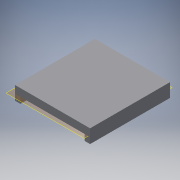
# Autodesk Inventor part: left gun mount
Saved by Autodesk Inventor 2018 (Build 220112000, 112)
## iProperties
Created: 2018-11-09
Part Number: left gun mount
Material: Generic
Document SubType Name: Modeling
Designer: Cameron
Mass: 123.699 g
Surface Area: 292.728 cm^2
Volume: 123.699 cm^3
Density: 1 g/cm^3
Appearance: Default
Author: Cameron
Autodesk Inventor part; units mm, degrees
ref_plane "YZ Plane" through (0, 0, 0) normal (1, 0, 0) x (0, 1, 0)
ref_plane "XZ Plane" through (0, 0, 0) normal (0, 1, 0) x (-1, 0, 0)
ref_plane "XY Plane" through (0, 0, 0) normal (0, 0, 1) x (1, 0, 0)
ref_plane "Work Plane1" through (0, 0, 0) normal (0, 0, 1) x (1, 0, 0)
sketch "Sketch1" plane through (0, 0, 0) normal (0, 0, 1) x (1, 0, 0)
  line L0 (4.5, 15) -> (-4.5, 15) projected
  line L1 (-4.5, 15) -> (-4.5, -15) projected
  line L2 (-4.5, -15) -> (4.5, -15) projected
  line L3 (4.5, -15) -> (4.5, -60.5) projected
  line L4 (4.5, -60.5) -> (89.5, -60.5) projected
  line L5 (89.5, -60.5) -> (89.5, 45) projected
  line L6 (89.5, 45) -> (4.5, 45) projected
  line L7 (4.5, 45) -> (4.5, 15) projected
  line L8 (96.5, 45) -> (-2.5, 45)
  line L9 (-2.5, 45) -> (-2.5, -60.5)
  line L10 (-2.5, -60.5) -> (96.5, -60.5)
  line L11 (96.5, -60.5) -> (96.5, 45)
  point P0 (0, 0)
  dimension "d0" = 7
  dimension "d1" = 7
  dimension "d2" = 0
  dimension "d3" = 0
  constraints: 8 end point, 2 parallel, 1 horizontal, 1 perpendicular
  measures "d0" distance between parallel lines of L11 L5
  measures "d1" distance between parallel lines of L9 L3
  measures "d2" distance between parallel lines of L10 L4
  measures "d3" distance between parallel lines of L8 L6
extrude "Extrusion1" add sketch "Sketch1" along normal blind 10 contours L7 L6 L5 L4 L3 L2 L9 L0 | L0 L9 L8 L7 | L2 L3 L10 L9 | L8 L11 L10 L5
sketch "Sketch2" plane through (0, 0, 0) normal (0, 0, -1) x (-1, 0, 0)
  line L0 (-96.5, -60.5) -> (-96.5, 45) projected
  line L1 (-96.5, 45) -> (2.5, 45) projected
  line L2 (2.5, -60.5) -> (-96.5, -60.5) projected
  line L3 (-69.73, -55.25) -> (-69.73, 39.65) projected
  line L4 (2.5, 45) -> (2.5, -60.5) projected
  line L5 (-4.5, 15) -> (4.5, 15) projected
  line L6 (4.5, 15) -> (4.5, -15) projected
  line L7 (4.5, -15) -> (-4.5, -15) projected
  line L8 (-4.5, -15) -> (-4.5, -60.5) projected
  line L9 (-4.5, -60.5) -> (-89.5, -60.5) projected
  line L10 (-89.5, -60.5) -> (-89.5, 45) projected
  line L11 (-89.5, 45) -> (-4.5, 45) projected
  line L12 (-4.5, 45) -> (-4.5, 15) projected
  line L13 (2.5, -60.5) -> (-96.5, -60.5) projected
  line L14 (-96.5, -60.5) -> (-89.5, -60.5)
  line L15 (-89.5, -60.5) -> (-89.5, 45)
  line L16 (-89.5, 45) -> (-96.5, 45)
  line L17 (-96.5, 45) -> (-96.5, -60.5)
  line L18 (-96.5, 45) -> (2.5, 45) projected
  line L19 (2.5, 45) -> (-4.5, 45)
  line L20 (-4.5, 45) -> (-4.5, 15)
  line L21 (-4.5, 15) -> (2.5, 15)
  line L22 (2.5, 15) -> (2.5, 45)
  line L23 (2.5, 45) -> (2.5, -60.5) projected
  line L24 (2.5, -15) -> (-4.5, -15)
  line L25 (-4.5, -15) -> (-4.5, -60.5)
  line L26 (-4.5, -60.5) -> (2.5, -60.5)
  line L27 (2.5, -60.5) -> (2.5, -15)
  point P0 (0, 0)
  dimension "d6" = 0
  constraints: 24 end point, 6 parallel, 3 horizontal, 3 perpendicular, 3 point on line
  measures "d6" distance between parallel lines of L25 L8
extrude "Extrusion2" add sketch "Sketch2" along normal blind 8 contours L0 L1 L10 L2 | L8 L7 L4 L2 | L1 L4 L5 L12
sketch "Sketch3" plane through (0, 0, 10) normal (0, 0, 1) x (1, 0, 0)
  line L0 (96.5, 45) -> (-2.5, 45) projected
  line L1 (-2.5, 45) -> (-2.5, -60.5) projected
  line L2 (-2.5, -60.5) -> (96.5, -60.5) projected
  line L3 (96.5, -60.5) -> (96.5, 45) projected
  circle A0 centre (47, -7.75) radius 25
  point P0 (0, 0)
  dimension "d9" = 50
  dimension "d10" = 49.5
  dimension "d11" = 49.5
  dimension "d12" = 52.75
  dimension "d13" = 52.75
  constraints: 1 centre point
  measures "d9" diameter of A0
  measures "d10" distance from line of L3 A0.centre
  measures "d11" distance from line of A0.centre L1
  measures "d12" distance from line of L2 A0.centre
  measures "d13" distance from line of L0 A0.centre
extrude "Extrusion3" add sketch "Sketch3" along normal blind 5 contours A0
sketch "Sketch4" plane through (47, -7.75, 15) normal (0, 0, 1) x (1, 0, 0)
  circle A0 centre (0, 0) radius 4 projected
  line L0 (3, -2.6458) -> (3, 2.6458) projected
  point P0 (-47, 7.75)
extrude "Extrusion4" cut sketch "Sketch4" against normal blind 20 contours L0 A0 picked at (-0.1458, -1.2472)
body "Solid1"
